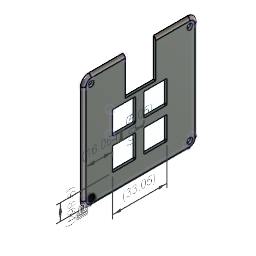
both (Autodesk Fusion 360 archive; units mm, degrees)
design "HackPad Upper case"
part number: 2026-02-04-21-46-16-954
Autodesk Fusion 360 part; units mm, degrees
sketch "plate-2026-02-04T20_06_32.880Z" plane through (0, 0, 0) normal (1, 0, 0) x (0, 1, 0)
  line L0 (5.0457, 37.2047) -> (18.0457, 37.2047)
  line L1 (5.0457, 23.2047) -> (18.0457, 23.2047)
  line L2 (4.5457, 36.7047) -> (4.5457, 23.7047)
  line L3 (18.5457, 36.7047) -> (18.5457, 23.7047)
  arc A0 (5.0457, 37.2047) -> (4.5457, 36.7047) centre (5.0457, 36.7047) ccw
  arc A1 (18.5457, 36.7047) -> (18.0457, 37.2047) centre (18.0457, 36.7047) ccw
  arc A2 (4.5457, 23.7047) -> (5.0457, 23.2047) centre (5.0457, 23.7047) ccw
  arc A3 (18.0457, 23.2047) -> (18.5457, 23.7047) centre (18.0457, 23.7047) ccw
  line L4 (24.0957, 37.2047) -> (37.0957, 37.2047)
  line L5 (24.0957, 23.2047) -> (37.0957, 23.2047)
  line L6 (23.5957, 36.7047) -> (23.5957, 23.7047)
  line L7 (37.5957, 36.7047) -> (37.5957, 23.7047)
  arc A4 (24.0957, 37.2047) -> (23.5957, 36.7047) centre (24.0957, 36.7047) ccw
  arc A5 (37.5957, 36.7047) -> (37.0957, 37.2047) centre (37.0957, 36.7047) ccw
  arc A6 (23.5957, 23.7047) -> (24.0957, 23.2047) centre (24.0957, 23.7047) ccw
  arc A7 (37.0957, 23.2047) -> (37.5957, 23.7047) centre (37.0957, 23.7047) ccw
  line L8 (5.0457, 18.1547) -> (18.0457, 18.1547)
  line L9 (5.0457, 4.1547) -> (18.0457, 4.1547)
  line L10 (4.5457, 17.6547) -> (4.5457, 4.6547)
  line L11 (18.5457, 17.6547) -> (18.5457, 4.6547)
  arc A8 (5.0457, 18.1547) -> (4.5457, 17.6547) centre (5.0457, 17.6547) ccw
  arc A9 (18.5457, 17.6547) -> (18.0457, 18.1547) centre (18.0457, 17.6547) ccw
  arc A10 (4.5457, 4.6547) -> (5.0457, 4.1547) centre (5.0457, 4.6547) ccw
  arc A11 (18.0457, 4.1547) -> (18.5457, 4.6547) centre (18.0457, 4.6547) ccw
  line L12 (24.0957, 18.1547) -> (37.0957, 18.1547)
  line L13 (24.0957, 4.1547) -> (37.0957, 4.1547)
  line L14 (23.5957, 17.6547) -> (23.5957, 4.6547)
  line L15 (37.5957, 17.6547) -> (37.5957, 4.6547)
  arc A12 (24.0957, 18.1547) -> (23.5957, 17.6547) centre (24.0957, 17.6547) ccw
  arc A13 (37.5957, 17.6547) -> (37.0957, 18.1547) centre (37.0957, 17.6547) ccw
  arc A14 (23.5957, 4.6547) -> (24.0957, 4.1547) centre (24.0957, 4.6547) ccw
  arc A15 (37.0957, 4.1547) -> (37.5957, 4.6547) centre (37.0957, 4.6547) ccw
sketch "Sketch2" plane through (0, 0, 0) normal (1, 0, 0) x (0, 1, 0)
sketch "Sketch3" plane through (0, 0, 0) normal (1, 0, 0) x (0, 1, 0)
  line L0 (-13.4543, -7.6453) -> (56.5457, -7.6453)
  line L1 (56.5457, -7.6453) -> (56.5457, 62.3547)
  line L2 (56.5457, 62.3547) -> (-13.4543, 62.3547)
  line L3 (-13.4543, 62.3547) -> (-13.4543, -7.6453)
  line L4 (12.2957, 62.3547) -> (30.7957, 62.3547)
  line L5 (30.7957, 62.3547) -> (30.7957, 39.3547)
  line L6 (30.7957, 39.3547) -> (12.2957, 39.3547)
  line L7 (12.2957, 39.3547) -> (12.2957, 62.3547)
  circle A0 centre (-8.4543, 57.3547) radius 1.7
  circle A1 centre (51.5457, 57.3547) radius 1.7
  circle A2 centre (51.5457, 57.3547) radius 1.7
  circle A3 centre (51.5457, 57.3547) radius 1.7
  circle A4 centre (51.5457, -2.6453) radius 1.7
  circle A5 centre (51.5457, -2.6453) radius 1.7
  circle A6 centre (-8.4543, -2.6453) radius 1.7
  dimension "d1" = 70
  dimension "d2" = 70
  dimension "d11" = 23
  dimension "d12" = 18.5
  dimension "d13" = 25.75
  dimension "d14" = 25.75
  dimension "d15" = 70
  dimension "d19" = 3.4
  dimension "d20" = 5
  dimension "d21" = 5
  dimension "d22" = 3.4
  dimension "d23" = 5
  dimension "d24" = 5
  dimension "d25" = 3.4
  dimension "d26" = 3.4
  dimension "d27" = 3.4
  dimension "d28" = 5
  dimension "d29" = 5
  dimension "d30" = 3.4
  dimension "d31" = 3.4
  dimension "d32" = 5
  constraint horizontal L0
  constraint vertical L1
  constraint horizontal L2
  constraint vertical L3
  constraint horizontal L4
  constraint vertical L5
  constraint horizontal L6
  constraint vertical L7
  constraint coincident L2 L4.start
  measures "d1" distance of L0.start L0.end
  measures "d2" distance of L0.start L2.end
  measures "d11" distance of L4.start L6.end
  measures "d12" distance of L5 L7
  measures "d13" distance of L3 L7
  measures "d14" distance of L1 L5
  measures "d15" distance of L1 L3
  measures "d19" diameter of A0
  measures "d20" distance of L2 A0.centre
  measures "d21" distance of L3 A0.centre
  measures "d22" diameter of A1
  measures "d23" distance of L2 A1.centre
  measures "d24" distance of L1 A1.centre
  measures "d25" diameter of A2
  measures "d26" diameter of A3
  measures "d27" diameter of A4
  measures "d28" distance of L0 A4.centre
  measures "d29" distance of L1 A4.centre
  measures "d30" diameter of A5
  measures "d31" diameter of A6
  measures "d32" distance of L3 A6.centre
extrude "Extrude1" add sketch "Sketch3" along normal blind 1.5 contours L0 L1 L2 L3 L5 L6 L7
extrude "Extrude2" cut sketch "plate-2026-02-04T20_06_32.880Z" along normal blind 0.5
delete_face "DeleteFace1" 1 faces at (0.5, 9.3791, 13.1547)
delete_face "DeleteFace2" 1 faces at (0.5, 9.3791, 27.8713)
delete_face "DeleteFace3" 1 faces at (0.5, 28.2624, 28.038)
delete_face "DeleteFace4" 1 faces at (0.5, 32.9291, 13.3213)
fillet "Fillet1" radius 5 4 edges at (0.75, -13.4543, -7.6453) (0.75, 56.5457, -7.6453) (0.75, 56.5457, 62.3547) (0.75, -13.4543, 62.3547)
fillet "Fillet2" radius 2 9 edges at (1.5, 1.9207, 62.3547) (1.5, -11.9898, 60.8902) (1.5, -13.4543, 27.3547) (1.5, -11.9898, -6.1809) (1.5, 21.5457, -7.6453) (1.5, 55.0813, -6.1809) (1.5, 56.5457, 27.3547) (1.5, 55.0813, 60.8902) (1.5, 41.1707, 62.3547)
sketch "Sketch4" plane through (0, 0, 0) normal (1, 0, 0) x (0, 1, 0)
  line L0 (-8.4543, 60.4182) -> (12.2957, 60.4182)
  line L1 (51.5457, -5.7089) -> (-8.4543, -5.7089)
  line L2 (4.5457, 36.7047) -> (4.5457, 23.7047)
  line L3 (-11.5178, -2.6453) -> (-11.5178, 57.3547)
  line L4 (54.6093, 57.3547) -> (54.6093, -2.6453)
  dimension "d41" = 66.127
  dimension "d42" = 16.0635
  dimension "d43" = 66.127
  measures "d41" distance of L0 L1
  measures "d42" distance of L2 L3
  measures "d43" distance of L3 L4
sketch "Sketch5" plane through (1.5, 0, 0) normal (1, 0, 0) x (0, 1, 0)
  line L0 (23.5957, 4.6547) -> (23.5957, 17.6547)
  arc A0 (24.0957, 18.1547) -> (23.5957, 17.6547) centre (24.0957, 17.6547) ccw
  line L1 (24.0957, 18.1547) -> (37.0957, 18.1547)
  arc A1 (37.5957, 17.6547) -> (37.0957, 18.1547) centre (37.0957, 17.6547) ccw
  line L2 (37.5957, 17.6547) -> (37.5957, 4.6547)
  arc A2 (37.0957, 4.1547) -> (37.5957, 4.6547) centre (37.0957, 4.6547) ccw
  line L3 (37.0957, 4.1547) -> (24.0957, 4.1547)
  arc A3 (23.5957, 4.6547) -> (24.0957, 4.1547) centre (24.0957, 4.6547) ccw
  line L4 (4.5457, 23.7047) -> (4.5457, 36.7047)
  arc A4 (5.0457, 37.2047) -> (4.5457, 36.7047) centre (5.0457, 36.7047) ccw
  line L5 (5.0457, 37.2047) -> (18.0457, 37.2047)
  arc A5 (18.5457, 36.7047) -> (18.0457, 37.2047) centre (18.0457, 36.7047) ccw
  line L6 (18.5457, 36.7047) -> (18.5457, 23.7047)
  arc A6 (18.0457, 23.2047) -> (18.5457, 23.7047) centre (18.0457, 23.7047) ccw
  line L7 (18.0457, 23.2047) -> (5.0457, 23.2047)
  arc A7 (4.5457, 23.7047) -> (5.0457, 23.2047) centre (5.0457, 23.7047) ccw
  line L8 (12.2957, 60.4182) -> (-8.4543, 60.4182)
  arc A8 (-8.4543, 60.4182) -> (-11.5178, 57.3547) centre (-8.4543, 57.3547) ccw
  line L9 (-11.5178, 57.3547) -> (-11.5178, -2.6453)
  arc A9 (-11.5178, -2.6453) -> (-8.4543, -5.7089) centre (-8.4543, -2.6453) ccw
  line L10 (-8.4543, -5.7089) -> (51.5457, -5.7089)
  arc A10 (51.5457, -5.7089) -> (54.6093, -2.6453) centre (51.5457, -2.6453) ccw
  line L11 (54.6093, -2.6453) -> (54.6093, 57.3547)
  arc A11 (54.6093, 57.3547) -> (51.5457, 60.4182) centre (51.5457, 57.3547) ccw
  line L12 (51.5457, 60.4182) -> (30.7957, 60.4182)
  line L13 (30.7957, 60.4182) -> (30.7957, 39.3547)
  line L14 (30.7957, 39.3547) -> (12.2957, 39.3547)
  line L15 (12.2957, 39.3547) -> (12.2957, 60.4182)
  circle A12 centre (51.5457, -2.6453) radius 1.7
  circle A13 centre (51.5457, 57.3547) radius 1.7
  circle A14 centre (-8.4543, 57.3547) radius 1.7
  circle A15 centre (-8.4543, -2.6453) radius 1.7
  line L16 (4.5457, 4.6547) -> (4.5457, 17.6547)
  arc A16 (5.0457, 18.1547) -> (4.5457, 17.6547) centre (5.0457, 17.6547) ccw
  line L17 (5.0457, 18.1547) -> (18.0457, 18.1547)
  arc A17 (18.5457, 17.6547) -> (18.0457, 18.1547) centre (18.0457, 17.6547) ccw
  line L18 (18.5457, 17.6547) -> (18.5457, 4.6547)
  arc A18 (18.0457, 4.1547) -> (18.5457, 4.6547) centre (18.0457, 4.6547) ccw
  line L19 (18.0457, 4.1547) -> (5.0457, 4.1547)
  arc A19 (4.5457, 4.6547) -> (5.0457, 4.1547) centre (5.0457, 4.6547) ccw
  line L20 (23.5957, 23.7047) -> (23.5957, 36.7047)
  arc A20 (24.0957, 37.2047) -> (23.5957, 36.7047) centre (24.0957, 36.7047) ccw
  line L21 (24.0957, 37.2047) -> (37.0957, 37.2047)
  arc A21 (37.5957, 36.7047) -> (37.0957, 37.2047) centre (37.0957, 36.7047) ccw
  line L22 (37.5957, 36.7047) -> (37.5957, 23.7047)
  arc A22 (37.0957, 23.2047) -> (37.5957, 23.7047) centre (37.0957, 23.7047) ccw
  line L23 (37.0957, 23.2047) -> (24.0957, 23.2047)
  arc A23 (23.5957, 23.7047) -> (24.0957, 23.2047) centre (24.0957, 23.7047) ccw
  circle A24 centre (-8.4543, -2.6453) radius 1.7
  dimension "d44" = 0
  dimension "d45" = 9.8635
  dimension "d46" = 16.0635
  dimension "d47" = 33.05
  dimension "d48" = 5.05
  dimension "d49" = 5.05
  measures "d45" distance of L10 L19
  measures "d46" distance of L9 L16
  measures "d47" distance of L2 L16
  measures "d48" distance of L0 L18
  measures "d49" distance of L7 L17
